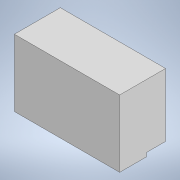
# Autodesk Inventor part: Apoio Motor
Saved by Autodesk Inventor 2021 (Build 250183000, 183)
## iProperties
Created: 2022-10-29
Part Number: Apoio Motor
Material: Genérico
Document SubType Name: Modeling
Designer: nicho
Density: 1 g/cm^3
Appearance: Padrão
Author: nicho
Autodesk Inventor part; units mm, degrees
ref_plane "YZ Plane" through (0, 0, 0) normal (1, 0, 0) x (0, 1, 0)
ref_plane "XZ Plane" through (0, 0, 0) normal (0, 1, 0) x (-1, 0, 0)
ref_plane "XY Plane" through (0, 0, 0) normal (0, 0, 1) x (1, 0, 0)
sketch "Esboço1" plane through (0, 0, 0) normal (1, 0, 0) x (0, 1, 0)
  line L0 (-17.5, 12) -> (17.5, 12)
  line L1 (17.5, 12) -> (17.5, -12)
  line L2 (17.5, -12) -> (-17.5, -12)
  line L3 (-17.5, -12) -> (-17.5, 12)
  line L4 (-17.5, 12) -> (17.5, -12) construction
  line L5 (17.5, 12) -> (-17.5, -12) construction
  point P0 (0, 0)
  dimension "d0" = 35
  dimension "d1" = 24
  constraints: 12 end point, 2 midpoint, 2 parallel, 1 horizontal, 1 perpendicular
  measures "d0" distance of L1.end L2.end
  measures "d1" distance of L0.end L1.end
extrude "Extrusão1" add sketch "Esboço1" along normal blind 55
sketch "Esboço2" plane through (0, -17.5, -12) normal (0, -1, 0) x (1, 0, 0)
  line L0 (55, 0) -> (55, 24) projected
  line L1 (0, 0) -> (55, 0)
  line L2 (55, 0) -> (55, 10)
  line L3 (55, 10) -> (0, 10)
  line L4 (0, 10) -> (0, 0)
  point P0 (0, 12)
  dimension "d4" = 10
  constraints: 8 end point, 2 parallel, 1 horizontal, 1 perpendicular, 1 point on line
  measures "d4" distance of L2.end L1.end
extrude "Extrusão2" cut sketch "Esboço2" against normal blind 2
